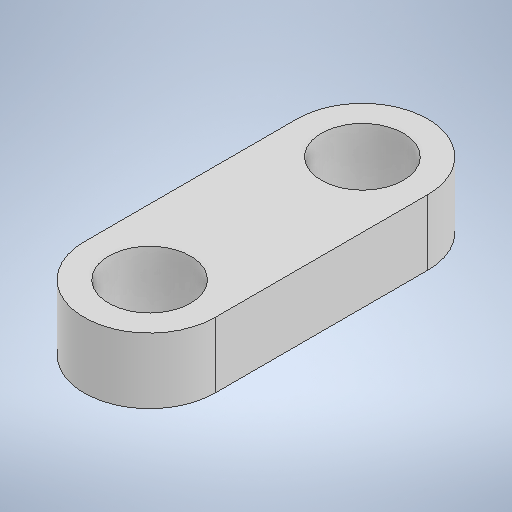
# Autodesk Inventor part: 12
Saved by Autodesk Inventor 2025.1 (Build 291241000, 241)
## iProperties
Created: 2024-09-13
Part Number: 12
Material: Generisch
Document SubType Name: Modeling
Designer: ffogue
Density: 1 g/cm^3
Appearance: Vorgabe
Author: ffogue
Autodesk Inventor part; units mm, degrees
ref_plane "YZ Plane" through (0, 0, 0) normal (1, 0, 0) x (0, 1, 0)
ref_plane "XZ Plane" through (0, 0, 0) normal (0, 1, 0) x (-1, 0, 0)
ref_plane "XY Plane" through (0, 0, 0) normal (0, 0, 1) x (1, 0, 0)
sketch "Sketch1" plane through (0, 0, 0) normal (0, 0, 1) x (1, 0, 0)
  line L0 (0, 6.5) -> (0, -6.5) construction
  line L1 (4, 6.5) -> (4, -6.5)
  line L2 (-4, -6.5) -> (-4, 6.5)
  arc A0 (4, 6.5) -> (-4, 6.5) centre (0, 6.5) ccw
  arc A1 (-4, -6.5) -> (4, -6.5) centre (0, -6.5) ccw
  point P0 (0, 0)
  point P1 (0, 0)
  dimension "d0" = 13
  dimension "d1" = 8
  constraints: 8 end point, 4 point on circle, 4 tangent, 2 centre point, 1 coincident, 1 midpoint, 1 parallel, 1 vertical
  measures "d0" distance of L0.start L0.end
  measures "d1" distance between parallel lines of L1 L2
extrude "Extrusion1" add sketch "Sketch1" along normal mid plane 4
sketch "Sketch2" plane through (0, 0, 2) normal (0, 0, 1) x (1, 0, 0)
  arc A0 (4, 6.5) -> (-4, 6.5) centre (0, 6.5) ccw projected
  arc A1 (-4, -6.5) -> (4, -6.5) centre (0, -6.5) ccw projected
  point P0 (0, 0)
  point P1 (0, 6.5)
  point P2 (0, -6.5)
  constraints: 2 coincident
hole "Hole1" at (0, 6.5, 2) at (0, -6.5, 2) direction (0, 0, -1) diameter 5 depth 4
body "Solid1"
